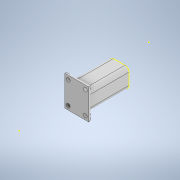
# Autodesk Inventor part: hank turn arm - connection
Saved by Autodesk Inventor 2022 (Build 260153000, 153)
## iProperties
Created: 2021-02-23
Part Number: hank turn arm - connection
Material: Generic
Document SubType Name: Modeling
Designer: chris
Density: 1 g/cm^3
Appearance: Default
Author: chris
Autodesk Inventor part; units mm, degrees
ref_plane "YZ Plane" through (0, 0, 0) normal (1, 0, 0) x (0, 1, 0)
ref_plane "XZ Plane" through (0, 0, 0) normal (0, 1, 0) x (-1, 0, 0)
ref_plane "XY Plane" through (0, 0, 0) normal (0, 0, 1) x (1, 0, 0)
sketch "Sketch1" plane through (0, 0, 0) normal (0, 0, 1) x (1, 0, 0)
  line L0 (-7.747, 7.747) -> (-7.747, -7.747)
  line L1 (-7.747, -7.747) -> (7.747, -7.747)
  line L2 (7.747, -7.747) -> (7.747, 7.747)
  line L3 (7.747, 7.747) -> (-7.747, 7.747)
  point P0 (0, 0)
  point P1 (0, 7.747)
  point P2 (-7.747, 0)
  dimension "d0" = 15.494
  dimension "d1" = 15.494
  dimension "d2" = 15.494
  constraints: 8 end point, 2 midpoint, 2 perpendicular, 1 horizontal alignment, 1 vertical, 1 vertical alignment
  measures "d0" distance of L0.start L0.end
  measures "d1" distance of L0.end L1.end
  measures "d2" distance of L1.end L2.end
extrude "Extrusion1" add sketch "Sketch1" along normal blind 63.5
sketch "Sketch2" plane through (0, 0, 0) normal (0, 0, -1) x (-1, 0, 0)
  circle A0 centre (0, 0) radius 2.286
  dimension "d5" = 4.572
  constraints: 1 centre point, 1 coincident
  measures "d5" diameter of A0
extrude "Extrusion2" cut sketch "Sketch2" against normal blind 19.05
sketch "Sketch3" plane through (7.747, -7.747, 0) normal (1, 0, 0) x (0, 0, -1)
  line L0 (-63.5, 0) -> (-63.5, 15.494) projected
  line L1 (-63.5, 22.987) -> (-63.5, -7.493)
  line L2 (0, 0) -> (0, 15.494) projected
  line L3 (-63.5, 22.987) -> (-120.65, 22.987)
  line L4 (-120.65, 22.987) -> (-120.65, -7.493)
  line L5 (-120.65, -7.493) -> (-63.5, -7.493)
  line L6 (-112.395, 17.907) -> (-71.755, 17.907)
  line L7 (-112.395, 17.907) -> (-112.395, -2.413)
  line L8 (-112.395, -2.413) -> (-71.755, -2.413)
  line L9 (-71.755, -2.413) -> (-71.755, 17.907)
  line L10 (-92.075, -7.493) -> (-92.075, 22.987)
  circle A0 centre (-116.3828, 2.794) radius 1.9939
  line L11 (-92.075, 7.747) -> (-101.3679, 7.747)
  circle A1 centre (-116.3828, 12.7) radius 1.9939
  circle A2 centre (-67.7672, 2.794) radius 1.9939
  circle A3 centre (-67.7672, 12.7) radius 1.9939
  line L12 (-112.395, 7.747) -> (-118.395, 7.747)
  line L13 (-118.395, 7.747) -> (-118.395, 10.247)
  line L14 (-118.395, 10.247) -> (-112.395, 10.247)
  line L15 (-118.395, 7.747) -> (-118.395, 5.247)
  line L16 (-118.395, 5.247) -> (-112.395, 5.247)
  line L17 (-81.8771, -14.1255) -> (-41.8771, -14.1255)
  point P0 (0, 7.747)
  point P1 (-63.5, 7.747)
  point P2 (0, 7.747)
  point P3 (-120.65, 7.747)
  point P4 (-92.075, 17.907)
  dimension "d9" = 30.48
  dimension "d10" = 57.15
  dimension "d11" = 40.64
  dimension "d12" = 20.32
  dimension "d16" = 24.3078
  dimension "d17" = 4.953
  dimension "d18" = 3.9878
  dimension "d19" = 6
  dimension "d20" = 2.5
  dimension "d21" = 2.5
  dimension "d25" = 40
  constraints: 32 end point, 8 midpoint, 6 horizontal, 6 perpendicular, 4 centre point, 4 vertical, 3 symmetric about line, 2 horizontal alignment, 2 point on line, 2 vertical alignment, 3 other
  measures "d9" distance of L1.start L1.end
  measures "d10" distance of L1.start L3.end
  measures "d11" distance of L6.start L6.end
  measures "d12" distance of L6.start L7.end
  measures "d16" distance from line of L10 A0.centre
  measures "d17" distance from line of L11 A0.centre
  measures "d18" diameter of A0
  measures "d19" distance of L12.start L12.end
  measures "d20" distance of L12.end L13.end
  measures "d21" distance of L12.end L15.end
  measures "d25" distance of L17.start L17.end
extrude "Extrusion3" add sketch "Sketch3" against normal blind 25.4 contours L1 L5 L10 L8 L9 L6 L3 L0 | L5 L4 L3 L10 L6 L7 L14 L13 L15 L16 L8 | L16 L15 L12 L7 | L7 L12 L13 L14 | A0 | A1 | A2 | A3
extrude "Extrusion4" cut sketch "Sketch3" against normal blind 57.15 contours L16 L15 L12 L7 | L7 L12 L13 L14 | A0 | A1 | A2 | A3
sketch "Sketch4" plane through (0, 0, 0) normal (0, 0, -1) x (-1, 0, 0)
  circle A0 centre (0, 0) radius 2.286 projected
  line L0 (7.747, 7.747) -> (7.747, -7.747) projected
  line L1 (-7.747, 7.747) -> (7.747, 7.747) projected
  line L2 (-7.747, -7.747) -> (-7.747, 7.747) projected
  line L3 (7.747, -7.747) -> (-7.747, -7.747) projected
sketch "Sketch5" plane through (7.747, -15.24, 120.65) normal (0, 0, 1) x (1, 0, 0)
  line L0 (0, 17.74) -> (-25.4, 17.74) projected
  line L1 (0, 25.4) -> (-25.4, 25.4) projected
  line L2 (0, 8.2931) -> (-25.4, 8.2931) projected
  line L3 (-25.4, 0) -> (-25.4, 30.48) projected
  line L4 (0, 0) -> (-25.4, 0) projected
  line L5 (0, 30.48) -> (0, 0) projected
  line L6 (0, 30.48) -> (-25.4, 30.48) projected
  point P0 (-7.747, 15.24)
extrude "Extrusion6" cut sketch "Sketch5" against normal blind 8.255
sketch "Sketch6" plane through (-17.653, -7.747, 0) normal (-1, 0, 0) x (0, 0, 1)
  circle A0 centre (67.7672, 2.794) radius 1.9939 projected
  circle A1 centre (67.7672, 12.7) radius 1.9939 projected
  line L0 (112.395, -7.493) -> (112.395, -2.413) projected
  line L1 (112.395, -2.413) -> (71.755, -2.413) projected
  line L2 (71.755, -2.413) -> (71.755, 17.907) projected
  line L3 (71.755, 17.907) -> (112.395, 17.907) projected
  line L4 (112.395, 17.907) -> (112.395, 22.987) projected
  line L5 (112.395, 22.987) -> (63.5, 22.987) projected
  line L6 (63.5, 22.987) -> (63.5, -7.493) projected
  line L7 (63.5, -7.493) -> (112.395, -7.493) projected
  point P0 (0, 7.747)
extrude "Extrusion7" cut sketch "Sketch6" against normal up to surface (9.906 mm away) contours A0 | A1 | L7 L6 L5 L4 L3 L2 L1 L0
sketch "Sketch7" plane through (-7.747, -7.747, 0) normal (-1, 0, 0) x (0, 0, 1)
  circle A0 centre (67.7672, 12.7) radius 1.9939 projected
  circle A1 centre (67.7672, 2.794) radius 1.9939 projected
  line L0 (0, 15.494) -> (0, 0) projected
  line L1 (0, 0) -> (63.5, 0) projected
  line L2 (63.5, -7.493) -> (63.5, 0) projected
  line L3 (112.395, -7.493) -> (63.5, -7.493) projected
  line L4 (112.395, -2.413) -> (112.395, -7.493) projected
  line L5 (71.755, -2.413) -> (112.395, -2.413) projected
  line L6 (71.755, 17.907) -> (71.755, -2.413) projected
  line L7 (112.395, 17.907) -> (71.755, 17.907) projected
  line L8 (112.395, 22.987) -> (112.395, 17.907) projected
  line L9 (63.5, 22.987) -> (112.395, 22.987) projected
  line L10 (63.5, 15.494) -> (63.5, 22.987) projected
  line L11 (0, 15.494) -> (63.5, 15.494) projected
  line L12 (0, 15.494) -> (63.5, 15.494) projected
  line L13 (0, 0) -> (63.5, 0) projected
  line L14 (63.5, 15.494) -> (63.5, 0)
  point P0 (0, 7.747)
  constraints: 2 end point, 1 vertical
extrude "Extrusion8" add sketch "Sketch7" along normal blind 4.953 contours L10 L9 L8 L7 L6 L5 L4 L3 L2 L14
mirror "Mirror1" about plane through (0, 0, 0) normal (1, 0, 0) of "Extrusion8"
fillet "Fillet4" radius 3.175 12 edges at (12.7, -15.24, 87.9475) (-12.7, -15.24, 87.9475) (12.7, 15.24, 87.9475) (-12.7, 15.24, 87.9475) (0, 15.24, 63.5) (-12.7, 0, 63.5) (0, -15.24, 63.5) (12.7, 0, 63.5) (-7.747, -7.747, 31.75) (-7.747, 7.747, 31.75) (7.747, -7.747, 31.75) (7.747, 7.747, 31.75)
sketch "Sketch9" plane through (0, 0, 0) normal (0, 0, -1) x (-1, 0, 0)
  circle A0 centre (0, 0) radius 2.286 projected
  arc A1 (7.747, 4.572) -> (4.572, 7.747) centre (4.572, 4.572) ccw projected
  line L0 (-4.572, 7.747) -> (4.572, 7.747) projected
  arc A2 (-4.572, 7.747) -> (-7.747, 4.572) centre (-4.572, 4.572) ccw projected
  line L1 (-7.747, -4.572) -> (-7.747, 4.572) projected
  arc A3 (-7.747, -4.572) -> (-4.572, -7.747) centre (-4.572, -4.572) ccw projected
  line L2 (4.572, -7.747) -> (-4.572, -7.747) projected
  arc A4 (4.572, -7.747) -> (7.747, -4.572) centre (4.572, -4.572) ccw projected
  line L3 (7.747, 4.572) -> (7.747, -4.572) projected
  circle A5 centre (0, 0) radius 2.286 projected
  circle A6 centre (0, 0) radius 2.6987
  dimension "d57" = 5.3975
  constraints: 1 centre point, 1 coincident
  measures "d57" diameter of A6
extrude "Extrusion9" cut sketch "Sketch9" against normal blind 33.02 contours A0 | L3 A4 L2 A3 L1 A2 L0 A1 | A6
extrude "Extrusion10" cut sketch "Sketch9" against normal blind 58.42 contours A0 | A6
sketch "Sketch10" plane through (-9.525, -15.24, 112.395) normal (0, -1, 0) x (1, 0, 0)
  line L0 (19.05, 0) -> (0, 0) projected
  line L1 (9.525, 0) -> (9.525, -6.35)
  circle A0 centre (3.937, -6.35) radius 1.9939
  circle A1 centre (15.113, -6.35) radius 1.9939
  point P0 (9.525, -112.395)
  dimension "d40" = 6.35
  dimension "d41" = 3.9878
  dimension "d42" = 5.588
  constraints: 2 centre point, 2 end point, 1 midpoint, 1 symmetric about line, 1 vertical, 1 other
  measures "d40" distance of L1.start L1.end
  measures "d41" diameter of A0
  measures "d42" distance of L1.end A0.centre
extrude "Extrusion11" cut sketch "Sketch10" against normal blind 3.175
mirror "Mirror2" about plane through (0, 0, 0) normal (0, 1, 0) of "Extrusion11"
sketch "Sketch11" plane through (-9.525, -15.24, 112.395) normal (0, -1, 0) x (1, 0, 0)
  circle A0 centre (3.937, -6.35) radius 1.9939 projected
  circle A1 centre (15.113, -6.35) radius 1.9939 projected
  line L0 (19.05, 0) -> (19.05, -45.72) projected
  line L1 (19.05, 0) -> (0, 0) projected
  line L2 (0, -45.72) -> (0, 0) projected
  line L3 (19.05, -45.72) -> (0, -45.72) projected
  circle A2 centre (9.525, -8.3458) radius 2
  line L4 (-3.175, -35.56) -> (22.225, -35.56) projected
  circle A3 centre (3.937, -35.56) radius 2
  circle A4 centre (9.525, -27.2053) radius 2
  circle A5 centre (15.113, -35.56) radius 2
  line L5 (10.525, -8.3458) -> (10.525, -27.2053)
  line L6 (8.525, -8.3458) -> (8.525, -27.2053)
  line L7 (3.1058, -35.004) -> (8.6938, -26.6494)
  line L8 (4.7682, -36.116) -> (10.3562, -27.7613)
  line L9 (9.525, -27.2053) -> (9.525, -20.7241)
  line L10 (15.9442, -35.004) -> (10.3562, -26.6494)
  line L11 (14.2818, -36.116) -> (8.6938, -27.7613)
  line L12 (3.9869, -20.7241) -> (0.7819, -18.9313)
  line L13 (0.7819, -18.9313) -> (0.7319, -15.2592)
  line L14 (0.7319, -15.2592) -> (3.8871, -13.3799)
  line L15 (3.8871, -13.3799) -> (7.0921, -15.1727)
  line L16 (7.0921, -15.1727) -> (7.1421, -18.8448)
  line L17 (7.1421, -18.8448) -> (3.9869, -20.7241)
  line L18 (15.0631, -20.7241) -> (18.2681, -18.9313)
  line L19 (18.2681, -18.9313) -> (18.3181, -15.2592)
  line L20 (18.3181, -15.2592) -> (15.1629, -13.3799)
  line L21 (15.1629, -13.3799) -> (11.9579, -15.1727)
  line L22 (11.9579, -15.1727) -> (11.9079, -18.8448)
  line L23 (11.9079, -18.8448) -> (15.0631, -20.7241)
  point P0 (9.525, -112.395)
  point P1 (3.937, -17.052)
  point P2 (15.113, -17.052)
  point P3 (5.7312, -34.6763)
  point P4 (9.525, -29.004)
  point P5 (13.3188, -34.6763)
  point P6 (14.9813, -33.5643)
  point P7 (11.3192, -28.0891)
  point P8 (10.525, -25.4733)
  point P9 (10.525, -10.0779)
  point P10 (8.525, -10.0779)
  point P11 (8.525, -25.4733)
  point P12 (7.7308, -28.0891)
  point P13 (4.0687, -33.5643)
  point P14 (9.6567, -29.201)
  point P15 (9.3933, -29.201)
  dimension "d45" = 4
  dimension "d46" = 4
  dimension "d47" = 4
  dimension "d48" = 4
  dimension "d49" = 18.8595
  constraints: 38 end point, 11 symmetric about line, 4 centre point, 1 point on line, 1 vertical, 13 other
  measures "d45" diameter of A2
  measures "d46" diameter of A3
  measures "d47" diameter of A4
  measures "d48" diameter of A5
  measures "d49" distance of L9.start A2.centre
extrude "Extrusion12" cut sketch "Sketch11" against normal blind 1 contours A5 L4 | L4 L11 A5 | L4 A5 L11 | A5 L11 A4 L10 | A3 L8 L4 | L4 A3 | L10 L5 A4 | A4 L11 L8 L7 L6 L5 L10 | L4 L8 A3 | L7 A4 L8 A3 | A4 L8 L11 | A4 L6 L7 | A4 L6 A2 L5 | A2 | L12 L13 L14 L15 L16 L17 | L23 L22 L21 L20 L19 L18
mirror "Mirror3" about plane through (0, 0, 0) normal (0, 1, 0) of "Extrusion12"
sketch "Sketch12" plane through (-9.525, -15.24, 112.395) normal (0, -1, 0) x (1, 0, 0)
  line L0 (-3.175, 0) -> (12.065, 0)
  line L1 (19.05, 0) -> (0, 0) projected
  arc A0 (9.3933, -29.201) -> (9.6567, -29.201) centre (9.525, -27.2053) ccw projected
  line L2 (9.3933, -29.201) -> (5.7312, -34.6763) projected
  arc A1 (4.0687, -33.5643) -> (5.7312, -34.6763) centre (3.937, -35.56) ccw projected
  line L3 (4.0687, -33.5643) -> (7.7308, -28.0891) projected
  arc A2 (8.525, -25.4733) -> (7.7308, -28.0891) centre (9.525, -27.2053) ccw projected
  line L4 (8.525, -25.4733) -> (8.525, -10.0779) projected
  arc A3 (10.525, -10.0779) -> (8.525, -10.0779) centre (9.525, -8.3458) ccw projected
  line L5 (10.525, -10.0779) -> (10.525, -25.4733) projected
  arc A4 (11.3192, -28.0891) -> (10.525, -25.4733) centre (9.525, -27.2053) ccw projected
  line L6 (11.3192, -28.0891) -> (14.9813, -33.5643) projected
  arc A5 (13.3188, -34.6763) -> (14.9813, -33.5643) centre (15.113, -35.56) ccw projected
  line L7 (13.3188, -34.6763) -> (9.6567, -29.201) projected
  line L8 (3.8871, -13.3799) -> (7.0921, -15.1727) projected
  line L9 (7.0921, -15.1727) -> (7.1421, -18.8448) projected
  line L10 (7.1421, -18.8448) -> (3.9869, -20.7241) projected
  line L11 (3.9869, -20.7241) -> (0.7819, -18.9313) projected
  line L12 (0.7819, -18.9313) -> (0.7319, -15.2592) projected
  line L13 (0.7319, -15.2592) -> (3.8871, -13.3799) projected
  line L14 (18.3181, -15.2592) -> (18.2681, -18.9313) projected
  line L15 (18.2681, -18.9313) -> (15.0631, -20.7241) projected
  line L16 (15.0631, -20.7241) -> (11.9079, -18.8448) projected
  line L17 (11.9079, -18.8448) -> (11.9579, -15.1727) projected
  line L18 (11.9579, -15.1727) -> (15.1629, -13.3799) projected
  line L19 (15.1629, -13.3799) -> (18.3181, -15.2592) projected
  circle A6 centre (3.937, -6.35) radius 1.9939 projected
  circle A7 centre (15.113, -6.35) radius 1.9939 projected
  line L20 (19.05, 0) -> (19.05, -45.72) projected
  line L21 (19.05, 0) -> (0, 0) projected
  line L22 (0, -45.72) -> (0, 0) projected
  line L23 (19.05, -45.72) -> (0, -45.72) projected
  line L24 (9.525, 0) -> (9.525, 9.5068)
  circle A8 centre (3.937, -6.35) radius 1.9939 projected
  line L25 (5.9309, -6.35) -> (7.0228, -6.35)
  point P0 (9.525, -112.395)
  dimension "d56" = 15.24
  constraints: 6 end point, 1 horizontal, 1 horizontal alignment, 1 midpoint, 1 point on line, 1 vertical, 1 other
  measures "d56" distance of L0.start L0.end
sketch "Sketch14" plane through (7.747, -15.24, 112.395) normal (0, 0, 1) x (1, 0, 0)
  line L0 (-34.0721, -11.2997) -> (-26.7755, 71.3954)
  line L1 (-26.7755, 71.3954) -> (24.444, 47.6456)
  line L2 (24.444, 47.6456) -> (16.8686, -15.7945)
  line L3 (16.8686, -15.7945) -> (-34.0721, -11.2997)
  point P0 (-7.747, 15.24)
  constraints: 8 end point, 1 perpendicular
sketch "Sketch15" plane through (9.525, -12.065, 63.5) normal (0, 0, -1) x (-1, 0, 0)
  line L0 (4.953, 19.812) -> (14.097, 19.812) projected
  arc A0 (17.272, 16.637) -> (14.097, 19.812) centre (14.097, 16.637) ccw projected
  line L1 (17.272, 7.493) -> (17.272, 16.637) projected
  arc A1 (14.097, 4.318) -> (17.272, 7.493) centre (14.097, 7.493) ccw projected
  line L2 (14.097, 4.318) -> (4.953, 4.318) projected
  arc A2 (1.778, 7.493) -> (4.953, 4.318) centre (4.953, 7.493) ccw projected
  line L3 (1.778, 16.637) -> (1.778, 7.493) projected
  arc A3 (4.953, 19.812) -> (1.778, 16.637) centre (4.953, 16.637) ccw projected
  line L4 (19.05, 0) -> (0, 0) projected
  line L5 (19.05, 24.13) -> (19.05, 0) projected
  line L6 (0, 24.13) -> (19.05, 24.13) projected
  line L7 (0, 0) -> (0, 24.13) projected
  line L8 (22.225, 22.225) -> (-3.175, 22.225) projected
  circle A4 centre (16.3421, 21.0176) radius 1.524
  circle A5 centre (2.7079, 21.0176) radius 1.524
  line L9 (22.225, 1.905) -> (22.225, 22.225) projected
  line L10 (22.225, 12.065) -> (19.05, 12.065)
  line L11 (19.05, 24.13) -> (19.05, 0) projected
  circle A6 centre (16.3421, 3.1124) radius 1.524
  circle A7 centre (2.7079, 3.1124) radius 1.524
  point P0 (9.525, 12.065)
  point P1 (15.4121, 22.225)
  point P2 (17.272, 22.225)
  dimension "d61" = 3.048
  dimension "d62" = 3.048
  constraints: 4 centre point, 2 end point, 2 midpoint, 2 symmetric about line, 2 other
  measures "d61" diameter of A4
  measures "d62" diameter of A5
extrude "Extrusion14" cut sketch "Sketch15" against normal blind 6.35 contours A5 L8 | L8 A5 | A4 L8 | L8 A4 | A6 | A7
sketch "Sketch16" plane through (0, 0, 33.02) normal (0, 0, -1) x (-1, 0, 0)
  circle A0 centre (0, 0) radius 2.6987 projected
  line L0 (7.747, 4.572) -> (7.747, -4.572) projected
  arc A1 (7.747, 4.572) -> (4.572, 7.747) centre (4.572, 4.572) ccw projected
  line L1 (-4.572, 7.747) -> (4.572, 7.747) projected
  arc A2 (-4.572, 7.747) -> (-7.747, 4.572) centre (-4.572, 4.572) ccw projected
  line L2 (-7.747, -4.572) -> (-7.747, 4.572) projected
  arc A3 (-7.747, -4.572) -> (-4.572, -7.747) centre (-4.572, -4.572) ccw projected
  line L3 (4.572, -7.747) -> (-4.572, -7.747) projected
  arc A4 (4.572, -7.747) -> (7.747, -4.572) centre (4.572, -4.572) ccw projected
sketch "Sketch17" plane through (7.747, -15.24, 112.395) normal (0, 0, 1) x (1, 0, 0)
  point P0 (-7.747, 15.24)
extrude "Extrusion16" cut sketch "Sketch14" against normal blind 46.99
sketch "Sketch18" plane through (9.525, -12.065, 63.5) normal (0, 0, -1) x (-1, 0, 0)
  line L0 (21.9599, 0) -> (21.9599, 24.13) projected
  line L1 (21.9599, 24.13) -> (19.05, 24.13) projected
  line L2 (19.05, 24.13) -> (19.05, 0) projected
  line L3 (19.05, 0) -> (21.9599, 0) projected
  arc A0 (19.05, -2.9099) -> (21.9599, 0) centre (19.05, 0) ccw projected
  arc A1 (19.05, -2.9099) -> (21.9599, 0) centre (19.05, 0) ccw projected
  line L4 (19.05, 0) -> (21.9599, 0) projected
  line L5 (19.05, -2.9099) -> (19.05, 0) projected
  line L6 (0, -2.9099) -> (19.05, -2.9099) projected
  line L7 (19.05, -2.9099) -> (19.05, 0) projected
  line L8 (19.05, 0) -> (0, 0) projected
  line L9 (0, 0) -> (0, -2.9099) projected
  arc A2 (-2.9099, 0) -> (0, -2.9099) centre (0, 0) ccw projected
  line L10 (0, 0) -> (0, -2.9099) projected
  line L11 (-2.9099, 0) -> (0, 0) projected
  line L12 (-2.9099, 24.13) -> (-2.9099, 0) projected
  line L13 (-2.9099, 0) -> (0, 0) projected
  line L14 (0, 0) -> (0, 24.13) projected
  line L15 (0, 24.13) -> (-2.9099, 24.13) projected
  line L16 (19.05, 27.0399) -> (0, 27.0399) projected
  line L17 (0, 27.0399) -> (0, 24.13) projected
  line L18 (0, 24.13) -> (19.05, 24.13) projected
  line L19 (19.05, 24.13) -> (19.05, 27.0399) projected
  arc A3 (21.9599, 24.13) -> (19.05, 27.0399) centre (19.05, 24.13) ccw projected
  line L20 (19.05, 24.13) -> (19.05, 27.0399) projected
  line L21 (21.9599, 24.13) -> (19.05, 24.13) projected
  arc A4 (0, 27.0399) -> (-2.9099, 24.13) centre (0, 24.13) ccw projected
  line L22 (0, 24.13) -> (-2.9099, 24.13) projected
  line L23 (0, 27.0399) -> (0, 24.13) projected
  point P0 (9.525, 12.065)
  point P1 (19.05, 24.13)
  point P2 (19.05, -2.9099)
  point P3 (0, 27.0399)
extrude "Extrusion17" cut sketch "Sketch18" against normal blind 46.99 contours L3 L2 L1 L0 | A0 L5 L3 | L1 L19 A3 | L5 L6 L9 L8 | L18 L17 L16 L19 | L9 A2 L11 | L11 L12 L15 L14 | L15 A4 L17
sketch "Sketch19" plane through (-9.525, -12.065, 63.5) normal (-1, 0, 0) x (0, 0, 1)
  point P0 (-63.5, 12.065)
sketch "Sketch20" plane through (7.747, -15.24, 65.405) normal (0, 0, 1) x (1, 0, 0)
  line L0 (1.778, 3.175) -> (1.778, 27.305) projected
  line L1 (1.778, 27.305) -> (-17.272, 27.305) projected
  line L2 (-17.272, 27.305) -> (-17.272, 3.175) projected
  line L3 (-17.272, 3.175) -> (1.778, 3.175) projected
  circle A0 centre (-0.9299, 6.2874) radius 1.524 projected
  circle A1 centre (-14.5641, 24.1926) radius 1.524 projected
  circle A2 centre (-14.5641, 6.2874) radius 1.524 projected
  circle A3 centre (-0.9299, 24.1926) radius 1.524 projected
  point P0 (-7.747, 15.24)
extrude "Extrusion18" add sketch "Sketch20" along normal blind 1.27
fillet "Fillet5" radius 3.175 4 edges at (0, -12.065, 63.5) (9.525, 0, 63.5) (-9.525, 0, 63.5) (0, 12.065, 63.5)
equation "\"d22\" = d10"
body "Solid1"
